Autodesk Fusion 360 part; units mm, degrees
(part 2 of 2)
  constraint concentric A17 A223
  constraint concentric A16 A224
  constraint concentric A15 A225
  constraint concentric A14 A226
  constraint concentric A13 A227
  constraint tangent A207 L200
  constraint tangent A206 L199
  constraint tangent A209 L202
  constraint tangent L198 A227
  constraint tangent L199 A207
  constraint tangent A219 L212
  constraint tangent A208 L201
  constraint tangent A225 L218
  constraint tangent A210 L203
  constraint tangent A211 L204
  constraint tangent A212 L205
  constraint tangent A213 L206
  constraint tangent L206 A214
  constraint tangent A218 L211
  constraint tangent A215 L208
  constraint tangent L208 A216
  constraint tangent A216 L209
  constraint tangent A217 L210
  constraint tangent A221 L214
  constraint tangent A220 L213
  constraint tangent A222 L215
  constraint tangent A223 L216
  constraint tangent A224 L217
  constraint tangent A226 L219
  constraint coincident L207 L243.start
  constraint coincident L241 L243.end
  constraint perpendicular L241 L243
  constraint coincident L208 L244.start
  constraint coincident L240 L244.end
  constraint perpendicular L240 L244
  constraint parallel L216 L245
  constraint tangent A246 L247
  constraint tangent A242 L248
  constraint tangent A241 L249
  constraint tangent L231 A251
  constraint tangent L232 A251
  constraint tangent L248 A252
  constraint tangent L249 A252
  constraint tangent L229 A253
  constraint tangent L230 A253
  constraint tangent L226 A254
  constraint tangent L227 A254
  constraint tangent L241 A255
  constraint tangent L242 A255
  constraint tangent L237 A256
  constraint tangent L238 A256
  constraint tangent L235 A257
  constraint tangent L236 A257
  constraint tangent L246 A258
  constraint tangent L247 A258
  constraint tangent L245 A259
  constraint tangent L246 A259
  constraint tangent L250 A260
  constraint tangent L250 A261
  constraint tangent L251 A262
  constraint tangent L251 A263
  measures "d1" diameter of A0
  measures "d2" diameter of A1
  measures "d3" diameter of A2
  measures "d4" diameter of A3
  measures "d5" diameter of A4
  measures "d9" diameter of A111
  measures "d12" diameter of A112
  measures "d305" diameter of A232
  measures "d306" diameter of A233
extrude "Extrude1" add sketch "mriya-bumper-sla" along normal blind 10.5 contours L198 A206 L199 A207 L200 A208 L201 A209 L202 A210 L203 A211 L204 A212 L205 A213 L206 A214 L207 L208 A216 L209 A217 L210 A218 L211 A219 L212 A220 L213 A221 L214 A222 L215 A223 L216 A224 L217 A225 L218 A226 L219 A227 A238 L226 L227 A239 L228 A240 L229 L230 A241 A242 L231 L232 A243 L233 A244 L234 A245 A246 L235 L236 A247 L237 L238 A248 L239 A249 L240 L241 L242 L243 L244 L245 L246 L247 L248 L249 A251 A252 A253 A254 A255 A256 A257 A258 A259 makes body 1
extrude "Extrude2" add sketch "mriya-bumper-sla" along normal blind 17 contours L207 A215 L208 L240 A250 L241 L243 L244 bodies 1
extrude "Extrude3" add sketch "mriya-bumper-sla" along normal blind 2 from surface at 1.7 contours A114 | A115 | A116 | A117 | L198 A206 L199 A207 L200 A208 L201 A209 L202 A210 L203 A211 L204 A212 L205 A213 L206 A214 L207 A215 L208 A216 L209 A217 L210 A218 L211 A219 L212 A220 L213 A221 L214 A222 L215 A223 L216 A224 L217 A225 L218 A226 L219 A227 L250 A260 A261 L251 A262 A263 | L207 L251 A262 A263 | L208 L250 A260 A261 | A232 | A233 bodies 1
extrude "Extrude6" add sketch "mriya-bumper-sla" along normal blind 1 from surface at 14.3 contours L207 L251 A262 A263 bodies 1
extrude "Extrude14" add sketch "mriya-bumper-sla" along normal blind 1 from surface at 7.7 contours L208 L250 A260 A261 bodies 1
extrude "Extrude15" cut sketch "mriya-bumper-sla" along normal blind 2.7 contours A232 | A233 bodies 1
chamfer "Chamfer8" distance 0.7 angle 45 2 edges at (-16.4, 78.0932, 14.3) (-7, 9.5932, 7.7) on bodies 1
sketch "power-switch" plane through (-4.4, 0, 0) normal (1, 0, 0) x (0, 1, 0)
  line L0 (36.0432, 5.4) -> (25.7432, 5.4)
  line L1 (25.7432, 5.4) -> (25.7432, 8.2)
  line L2 (25.7432, 8.2) -> (36.0432, 8.2)
  line L3 (36.0432, 8.2) -> (36.0432, 5.4)
  line L4 (36.4432, 4) -> (25.3432, 4)
  line L5 (24.3432, 5) -> (24.3432, 8.6)
  line L6 (25.3432, 9.6) -> (36.4432, 9.6)
  line L7 (37.4432, 8.6) -> (37.4432, 5)
  arc A0 (25.3432, 9.6) -> (24.3432, 8.6) centre (25.3432, 8.6) ccw
  arc A1 (37.4432, 8.6) -> (36.4432, 9.6) centre (36.4432, 8.6) ccw
  arc A2 (36.4432, 4) -> (37.4432, 5) centre (36.4432, 5) ccw
  arc A3 (24.3432, 5) -> (25.3432, 4) centre (25.3432, 5) ccw
  line L8 (1.9932, 0) -> (76.4932, 0)
  line L9 (76.4932, 0) -> (76.4932, 17)
  line L10 (76.4932, 17) -> (19.3932, 17)
  line L11 (19.3932, 17) -> (19.3932, 10.5)
  line L12 (19.3932, 10.5) -> (1.9932, 10.5)
  line L13 (1.9932, 10.5) -> (1.9932, 0)
  constraint perpendicular L0 L1
  constraint tangent L5 A0
  constraint tangent L6 A0
  constraint tangent L6 A1
  constraint tangent L7 A1
  constraint tangent L4 A2
  constraint tangent L7 A2
  constraint tangent L4 A3
  constraint tangent L5 A3
  constraint vertical L1
  constraint perpendicular L1 L2
  constraint vertical L3
extrude "Extrude8" cut sketch "power-switch" against normal blind 2.6 contours L0 L1 L2 L3 bodies 1
extrude "Extrude9" cut sketch "power-switch" against normal blind 1.2 contours L4 L5 L6 L7 A0 A1 A2 A3 bodies 1
chamfer "Chamfer9" distance 1.2 angle 45 8 edges at (-4.4, 30.8932, 4) (-4.4, 24.6361, 4.2929) (-4.4, 24.3432, 6.8) (-4.4, 24.6361, 9.3071) (-4.4, 30.8932, 9.6) (-4.4, 37.1503, 9.3071) (-4.4, 37.4432, 6.8) (-4.4, 37.1503, 4.2929) on bodies 1
sketch "usb-c" plane through (0, 80.6932, 0) normal (0, 1, 0) x (-1, 0, 0)
  line L0 (10.9002, 11.05) -> (10.9002, 10.15)
  arc A0 (21.0002, 11.05) -> (19.7002, 12.35) centre (19.7002, 11.05) ccw
  arc A1 (11.8003, 10.15) -> (13.1003, 8.85) centre (13.1002, 10.15) ccw
  line L1 (21.9002, 11.05) -> (21.9002, 10.15)
  line L2 (13.1002, 12.35) -> (19.7002, 12.35)
  line L3 (11.8003, 10.15) -> (11.8003, 11.05)
  line L4 (13.1002, 13.25) -> (19.7002, 13.25)
  line L5 (19.7002, 7.95) -> (13.1002, 7.95)
  arc A2 (13.1002, 12.35) -> (11.8003, 11.05) centre (13.1002, 11.05) ccw
  line L6 (19.7002, 8.85) -> (13.1002, 8.85)
  line L7 (21.0002, 11.05) -> (21.0002, 10.15)
  arc A3 (19.7002, 8.85) -> (21.0002, 10.15) centre (19.7003, 10.15) ccw
  arc A4 (13.1002, 13.25) -> (10.9002, 11.05) centre (13.1002, 11.05) ccw
  arc A5 (10.9002, 10.15) -> (13.1002, 7.95) centre (13.1002, 10.15) ccw
  arc A6 (21.9002, 11.05) -> (19.7003, 13.25) centre (19.7003, 11.05) ccw
  arc A7 (19.7002, 7.95) -> (21.9002, 10.15) centre (19.7002, 10.15) ccw
  line L8 (8.6, 0) -> (41.0674, 0)
  line L9 (41.0674, 0) -> (41.0674, 10.5)
  line L10 (41.0674, 10.5) -> (25.7, 10.5)
  line L11 (25.7, 10.5) -> (25.7, 17)
  line L12 (25.7, 17) -> (8.6, 17)
  line L13 (8.6, 17) -> (8.6, 0)
  constraint horizontal L5
  constraint tangent L3 A2
  constraint tangent L2 A2
  constraint tangent A1 L6
  constraint tangent A1 L3
  constraint tangent A0 L2
  constraint tangent A0 L7
  constraint tangent L7 A3
  constraint tangent L6 A3
  constraint parallel L1 L3
  constraint tangent L0 A4
  constraint tangent L4 A4
  constraint tangent L5 A5
  constraint tangent L0 A5
  constraint tangent L4 A6
  constraint tangent L1 A6
  constraint tangent L1 A7
  constraint tangent L5 A7
extrude "Extrude10" cut sketch "usb-c" against normal blind 2.6 contours A0 A1 L2 L3 A2 L6 L7 A3 bodies 1
extrude "Extrude11" cut sketch "usb-c" against normal blind 1.2 contours L0 L1 L4 L5 A4 A5 A6 A7 bodies 1
chamfer "Chamfer10" distance 1.2 angle 45 8 edges at (-16.4003, 80.6932, 7.95) (-11.5446, 80.6932, 8.5944) (-10.9003, 80.6932, 10.6) (-11.5446, 80.6932, 12.6056) (-16.4003, 80.6932, 13.25) (-21.2559, 80.6932, 12.6056) (-21.9003, 80.6932, 10.6) (-21.2559, 80.6932, 8.5944) on bodies 1
fillet "Fillet32" radius 0.6 4 edges at (-5.7, 19.3932, 10.5) (-5.7, 19.3932, 17) (-25.7, 79.3932, 10.5) (-25.7, 79.3932, 17) on bodies 1
fillet "Fillet33" radius 1.2 96 edges at (-16.85, 80.6932, 17) (-25.5243, 80.6932, 16.8243) (-25.7, 80.6932, 13.75) (-25.8757, 80.6932, 10.6757) (-33.6837, 80.6932, 10.5) (-41.4501, 80.7693, 10.5) (-42.0898, 81.3013, 10.5) (-43.9298, 82.6354, 10.5) (-51.7979, 82.9932, 10.5) (-58.2501, 83.0693, 10.5) (-59.9898, 84.7013, 10.5) (-62.9298, 87.1354, 10.5) (-73.4, 87.4932, 10.5) (-83.8702, 87.1354, 10.5) (-86.3102, 85.2013, 10.5) (-87.5499, 84.0693, 10.5) (-94.5021, 83.9932, 10.5) (-102.8702, 83.6354, 10.5) (-107.487, 79.5246, 10.5) (-111.0657, 76.1074, 10.5) (-115.8556, 75.9932, 10.5) (-121.8702, 75.6354, 10.5) (-123.7102, 74.3013, 10.5) (-124.3499, 73.7693, 10.5) (-131.4163, 73.6932, 10.5) (-141.0698, 72.463, 10.5) (-142.3, 42.8932, 10.5) (-141.0698, 13.3234, 10.5) (-120.6213, 12.0932, 10.5) (-100.9613, 12.5271, 10.5) (-96.1665, 16.7083, 10.5) (-92.7343, 19.979, 10.5) (-84.6934, 20.0932, 10.5) (-75.7143, 19.6842, 10.5) (-70.7197, 11.6751, 10.5) (-65.1018, 3.0339, 10.5) (-55.7327, 2.3932, 10.5) (-48.3499, 2.3171, 10.5) (-47.7102, 1.7851, 10.5) (-45.8702, 0.451, 10.5) (-36.9021, 0.0932, 10.5) (-29.3499, 0.0171, 10.5) (-28.7102, -0.5149, 10.5) (-26.8702, -1.849, 10.5) (-16.8358, -2.2068, 10.5) (-5.6302, -0.9766, 10.5) (-4.4, 10.3932, 10.5) (-4.4, 19.2175, 10.6757) (-4.4, 19.3932, 13.75) (-4.4, 19.5689, 16.8243) (-4.4, 48.2432, 17) (-5.6302, 79.463, 17) (-24.8337, 80.6932, 0) (-41.4501, 80.7693, 0) (-42.0898, 81.3013, 0) (-43.9298, 82.6354, 0) (-51.7979, 82.9932, 0) (-58.2501, 83.0693, 0) (-59.9898, 84.7013, 0) (-62.9298, 87.1354, 0) (-73.4, 87.4932, 0) (-83.8702, 87.1354, 0) (-86.3102, 85.2013, 0) (-87.5499, 84.0693, 0) (-94.5021, 83.9932, 0) (-102.8702, 83.6354, 0) (-107.487, 79.5246, 0) (-111.0657, 76.1074, 0) (-115.8556, 75.9932, 0) (-121.8702, 75.6354, 0) (-123.7102, 74.3013, 0) (-124.3499, 73.7693, 0) (-131.4163, 73.6932, 0) (-141.0698, 72.463, 0) (-142.3, 42.8932, 0) (-141.0698, 13.3234, 0) (-120.6213, 12.0932, 0) (-100.9613, 12.5271, 0) (-96.1665, 16.7083, 0) (-92.7343, 19.979, 0) (-84.6934, 20.0932, 0) (-75.7143, 19.6842, 0) (-70.7197, 11.6751, 0) (-65.1018, 3.0339, 0) (-55.7327, 2.3932, 0) (-48.3499, 2.3171, 0) (-47.7102, 1.7851, 0) (-45.8702, 0.451, 0) (-36.9021, 0.0932, 0) (-29.3499, 0.0171, 0) (-28.7102, -0.5149, 0) (-26.8702, -1.849, 0) (-16.8358, -2.2068, 0) (-5.6302, -0.9766, 0) (-4.4, 39.2432, 0) (-5.6302, 79.463, 0) on bodies 1
mirror "Mirror1" about plane through (0, 0, 0) normal (1, 0, 0) of bodies 1 makes body 2
named bodies: "Left", "Right"
